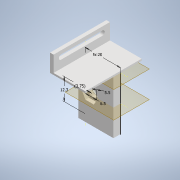
# Autodesk Inventor part: Enoder_Mount1
Saved by Autodesk Inventor 2022 (Build 260153000, 153)
## iProperties
Created: 2024-04-26
Part Number: Enoder_Mount1
Material: Generic
Document SubType Name: Modeling
Designer: raphael.hauk
Density: 1 g/cm^3
Appearance: Default
Author: raphael.hauk
Autodesk Inventor part; units mm, degrees
ref_plane "YZ Plane" through (0, 0, 0) normal (1, 0, 0) x (0, 1, 0)
ref_plane "XY Plane" through (0, 0, 0) normal (0, 0, 1) x (1, 0, 0)
ref_plane "MountingScrew" through (0, 0, 0) normal (0, 1, 0) x (-1, 0, 0)
ref_plane "Bracketheight" through (0, 15, 0) normal (0, 1, 0) x (-1, 0, 0)
sketch "Sketch1" plane through (0, 0, 0) normal (0, 0, 1) x (1, 0, 0)
  line L0 (0, -15.05) -> (20, -15.05)
  line L1 (20, -15.05) -> (20, 15)
  line L2 (20, 15) -> (0, 15)
  line L3 (0, 15) -> (0, -15.05)
  circle A0 centre (6, 0) radius 2.75 construction
  line L4 (0, -2.75) -> (20, -2.75) construction
  line L5 (3.25, 15) -> (3.25, -15.05) construction
  line L6 (-4, 0) -> (24, 0) construction
  line L7 (0, 21.01) -> (0, -21.06) construction
  line L8 (-4, 15) -> (24, 15) construction
  dimension "d0" = 5.5
  dimension "d1" = 12.3
  dimension "d2" = 3.25
  dimension "d31" = 6
  dimension "d36" = 20
  constraints: 12 end point, 7 point on line, 3 perpendicular, 2 parallel, 2 tangent, 1 centre point, 1 horizontal
  measures "d0" diameter of A0
  measures "d1" distance between parallel lines of L0 L4
  measures "d2" distance between parallel lines of L3 L5
  measures "d31" distance from line of L3 A0.centre
  measures "d36" distance of L1.end L2.end
extrude "Extrusion1" add sketch "Sketch1" along normal blind 4
sketch "Sketch2" plane through (0, 0, 4) normal (0, 0, 1) x (1, 0, 0)
  point P0 (0, 0)
  point P1 (6, 0)
hole "Hole1" at (6, 0, 4) direction (0, 0, -1) diameter 5.3 end through all clearance for "Socket Head Cap Screw ISO 4762" size "M5" standard "ISO"
sketch "Sketch5" plane through (0, 15, 0) normal (0, 1, 0) x (1, 0, 0)
  line L0 (0, 12) -> (20, 12)
  line L1 (20, 12) -> (20, -20)
  line L2 (20, -20) -> (0, -20)
  line L3 (0, -20) -> (0, 12)
  line L4 (20, 0) -> (0, 0) construction
  line L5 (20, 0) -> (0, 0) construction
  line L6 (0, 0) -> (0, -4) construction
  line L7 (20, 0) -> (20, -4) construction
  dimension "d2" = 3.25
  dimension "d60" = 20
  dimension "d61" = 12
  constraints: 8 end point, 2 midpoint, 2 parallel, 1 horizontal, 1 perpendicular
  measures "d60" distance between parallel lines of L2 L4
  measures "d61" distance between parallel lines of L0 L4
extrude "Extrusion4" add sketch "Sketch5" along normal blind 1
sketch "Sketch6" plane through (0, -15.05, 0) normal (-1, 0, 0) x (0, 0, 1)
  line L0 (-12, 30.05) -> (0, 30.05) projected
  line L1 (-12, 30.05) -> (20, 30.05)
  line L2 (20, 30.05) -> (20, 40.05)
  line L3 (20, 40.05) -> (-12, 40.05)
  line L4 (-12, 40.05) -> (-12, 30.05)
  line L5 (20, 30.05) -> (20, 31.05) construction
  point P0 (0, 15.05)
  dimension "d37" = 10
  constraints: 8 end point, 2 parallel, 1 horizontal, 1 perpendicular, 1 point on line
  measures "d37" distance of L1.end L2.end
extrude "Extrusion5" add sketch "Sketch6" against normal blind 2
sketch "Sketch8" plane through (5.5, 0, 4) normal (0, 0, 1) x (1, 0, 0)
  line L0 (-1.8671, 4.1) -> (2.8671, 4.1)
  line L1 (2.8671, 4.1) -> (5.2343, 0)
  line L2 (5.2343, 0) -> (2.8671, -4.1)
  line L3 (2.8671, -4.1) -> (-1.8671, -4.1)
  line L4 (-1.8671, -4.1) -> (-4.2343, 0)
  line L5 (-4.2343, 0) -> (-1.8671, 4.1)
  point P0 (-5.5, 0)
  point P1 (0.5, 0)
  point P2 (0.5, 0)
  dimension "d42" = 8.2
  constraints: 12 end point, 1 coincident, 1 horizontal, 13 other
  measures "d42" distance between parallel lines of L3 L0
extrude "Extrusion7" cut sketch "Sketch8" against normal blind 2
sketch "Sketch10" plane through (0, -15.05, 0) normal (-1, 0, 0) x (0, 0, 1)
  line L0 (-7.7, 36.75) -> (15.7, 36.75) construction
  line L1 (-7.7, 35.45) -> (15.7, 35.45)
  line L2 (15.7, 38.05) -> (-7.7, 38.05)
  arc A0 (-7.7, 38.05) -> (-7.7, 35.45) centre (-7.7, 36.75) ccw
  arc A1 (15.7, 35.45) -> (15.7, 38.05) centre (15.7, 36.75) ccw
  line L3 (-12, 30.05) -> (-12, 40.05) projected
  line L4 (0, 30.05) -> (0, 0) projected
  line L5 (0, 30.05) -> (0, 0) projected
  line L6 (20, 40.05) -> (-12, 40.05) projected
  line L7 (20, 30.05) -> (20, 40.05) projected
  point P0 (0, 15.05)
  point P1 (4, 36.75)
  point P2 (-12, 35.05)
  dimension "d55" = 2.6
  dimension "d59" = 2
  dimension "d63" = 4.3
  dimension "d64" = 4.3
  constraints: 8 end point, 4 point on circle, 4 tangent, 2 centre point, 2 midpoint, 1 horizontal, 1 parallel
  measures "d55" distance between parallel lines of L1 L2
  measures "d59" distance between parallel lines of L6 L2
  measures "d63" distance from line of L7 L0.end
  measures "d64" distance from line of L3 L0.start
extrude "Extrusion9" cut sketch "Sketch10" against normal through all
sketch "Sketch7" plane through (0, 15, 0) normal (0, -1, 0) x (1, 0, 0)
  line L0 (20, 4) -> (0, 4) projected
  line L1 (0, 4) -> (0, 20) projected
  line L2 (20, 4) -> (0, 4)
  line L3 (0, 4) -> (0, 20)
  line L4 (0, 20) -> (20, 20)
  line L5 (20, 20) -> (20, 4)
  point P0 (0, 0)
  dimension "d45" = 5.1
  dimension "d16" = 2.5
  dimension "d17" = 4.25
  dimension "d18" = 8
  constraints: 6 end point, 2 centre point, 2 point on circle, 2 point on line, 2 tangent, 1 coincident, 1 symmetric about line, 1 other
sketch "Sketch4" plane through (25.5, -5.5, 0) normal (1, 0, 0) x (0, 0, -1)
  line L0 (-5.45, 24.0278) -> (-8, 22.5555)
  line L1 (-8, 22.5555) -> (-10.55, 24.0278)
  line L2 (-10.55, 24.0278) -> (-10.55, 26.9722)
  line L3 (-10.55, 26.9722) -> (-8, 28.4445)
  line L4 (-8, 28.4445) -> (-5.45, 26.9722)
  line L5 (-5.45, 26.9722) -> (-5.45, 24.0278)
  point P0 (0, 5.5)
  point P1 (-8, 25.5)
  point P2 (-8, 25.5)
  dimension "d28" = 5.1
  constraints: 12 end point, 1 coincident, 1 vertical, 13 other
  measures "d28" distance between parallel lines of L5 L2
equation "\"d36\" = Schraubenlaenge"
equation "\"d64\" = d63"
equation "\"Schraubenlaenge\" = 20"
body "Solid1"
